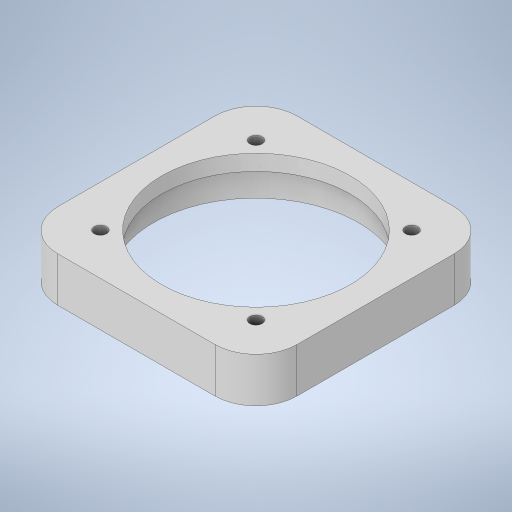
# Autodesk Inventor part: 사이클로이드 기어 하우징
Saved by Autodesk Inventor 2023 (Build 270158000, 158)
## iProperties
Created: 2022-06-19
Part Number: 사이클로이드 기어 하우징
Material: 일반
Document SubType Name: Modeling
Designer: fly01
Density: 1 g/cm^3
Appearance: 기본값
Author: fly01
Autodesk Inventor part; units mm, degrees
ref_plane "YZ Plane" through (0, 0, 0) normal (1, 0, 0) x (0, 1, 0)
ref_plane "XZ Plane" through (0, 0, 0) normal (0, 1, 0) x (-1, 0, 0)
ref_plane "XY Plane" through (0, 0, 0) normal (0, 0, 1) x (1, 0, 0)
sketch "스케치1" plane through (0, 0, 0) normal (0, 0, 1) x (1, 0, 0)
  line L0 (-25, -30) -> (25, -30) construction
  line L1 (30, -25) -> (30, 25) construction
  line L2 (25, 30) -> (-25, 30) construction
  line L3 (-30, 25) -> (-30, -25) construction
  line L4 (-30, -30) -> (30, 30) construction
  line L5 (30, -30) -> (-30, 30) construction
  arc A0 (-25, 30) -> (-30, 25) centre (-25, 25) ccw
  arc A1 (30, 25) -> (25, 30) centre (25, 25) ccw
  arc A2 (25, -30) -> (30, -25) centre (25, -25) ccw
  arc A3 (-30, -25) -> (-25, -30) centre (-25, -25) ccw
  circle A4 centre (0, 0) radius 7.5
  circle A5 centre (0, 0) radius 35 construction
  circle A6 centre (-24.7487, 24.7487) radius 2
  circle A7 centre (-24.7487, -24.7487) radius 2
  circle A8 centre (24.7487, -24.7487) radius 2
  circle A9 centre (24.7487, 24.7487) radius 2
  circle A10 centre (0, 0) radius 32.6
  circle A11 centre (0, 0) radius 25 construction
  line L6 (-25, 38) -> (25, 38)
  arc A12 (38, 25) -> (25, 38) centre (25, 25) ccw
  line L7 (38, 25) -> (38, -25)
  arc A13 (25, -38) -> (38, -25) centre (25, -25) ccw
  line L8 (25, -38) -> (-25, -38)
  arc A14 (-38, -25) -> (-25, -38) centre (-25, -25) ccw
  line L9 (-38, -25) -> (-38, 25)
  arc A15 (-25, 38) -> (-38, 25) centre (-25, 25) ccw
  dimension "d4" = 70
  dimension "d0" = 60
  dimension "d1" = 60
  dimension "d2" = 5
  dimension "d3" = 15
  dimension "d5" = 4
  dimension "d8" = 360
  dimension "d10" = 65.2
  dimension "d11" = 50
  dimension "d12" = 8
  constraints: 20 end point, 16 point on circle, 15 centre point, 9 point on line, 8 tangent, 4 coincident, 4 parallel, 3 equal radius, 2 midpoint, 2 perpendicular, 1 horizontal, 19 other
  measures "d0" distance of L5.end L4.end
  measures "d1" distance of L4.end L5.start
  measures "d2" radius of A0
  measures "d3" diameter of A4
  measures "d5" diameter of A6
  measures "d10" diameter of A10
  measures "d11" diameter of A11
  measures "d12" distance between parallel lines of L2 L6
extrude "돌출1" add sketch "스케치1" along normal blind 9.2 contours L6 A12 L7 A13 L8 A14 L9 A15
sketch "스케치2" plane through (0, 0, 0) normal (0, 0, -1) x (-1, 0, 0)
  line L0 (25, -38) -> (-25, -38) projected
  arc A0 (25, -38) -> (38, -25) centre (25, -25) ccw projected
  line L1 (38, 25) -> (38, -25) projected
  arc A1 (38, 25) -> (25, 38) centre (25, 25) ccw projected
  line L2 (-25, 38) -> (25, 38) projected
  arc A2 (-25, 38) -> (-38, 25) centre (-25, 25) ccw projected
  line L3 (-38, -25) -> (-38, 25) projected
  arc A3 (-38, -25) -> (-25, -38) centre (-25, -25) ccw projected
  circle A4 centre (0, 0) radius 32.6 construction
  circle A5 centre (-24.7487, 24.7487) radius 2 projected
  circle A6 centre (-24.7487, -24.7487) radius 2 projected
  circle A7 centre (24.7487, -24.7487) radius 2 projected
  circle A8 centre (24.7487, 24.7487) radius 2 projected
  circle A9 centre (0, 0) radius 30
  dimension "d15" = 60
  constraints: 1 centre point, 1 coincident
  measures "d15" diameter of A9
extrude "돌출2" add sketch "스케치2" along normal blind 5
